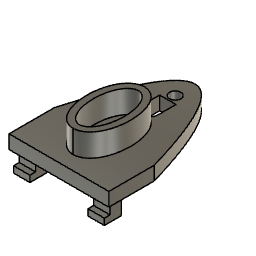
Here3 GPS Link Top Mount (Autodesk Fusion 360 design; units mm, degrees)
Autodesk Fusion 360 part; units mm, degrees
sketch "Sketch1" plane through (0, 0, 0) normal (0, 0, 1) x (1, 0, 0)
  line L0 (0, 0) -> (5.842, 0)
  line L1 (5.842, 0) -> (22.098, 0)
  line L2 (22.098, 0) -> (27.94, 0)
  line L3 (0, 0) -> (0, 12.7)
  line L4 (27.94, 0) -> (27.94, 12.7)
  line L5 (0, 0) -> (13.97, 0)
  line L6 (13.97, 0) -> (13.97, 38.1)
  spline S0 degree 5 poles (0, 12.7) (0.5588, 14.6265) (1.6764, 18.3113) (3.3528, 23.3339) (5.588, 29.0044) (8.382, 34.2662) (11.176, 37.5384) (13.97, 38.6587) (16.764, 37.5384) (19.558, 34.2662) (22.352, 29.0044) (24.5872, 23.3339) (26.2636, 18.3113) (27.3812, 14.6265) (27.94, 12.7) knots 0 0 0 0 0 0 0.1 0.2 0.3 0.4 0.5 0.6 0.7 0.8 0.9 1 1 1 1 1 1
  dimension "d1" = 5.842
  dimension "d2" = 16.256
  dimension "d3" = 5.842
  dimension "d28" = 13.97
  dimension "d29" = 38.1
  constraint coincident L0.start L3.start
  constraint horizontal L0
  constraint parallel L0 L1
  constraint parallel L1 L2
  constraint perpendicular L0 L3
  constraint perpendicular L2 L4
  constraint perpendicular L3 L5
  constraint perpendicular L5 L6
  measures "d1" distance of L0.start L0.end
  measures "d2" distance of L0.end L1.end
  measures "d3" distance of L1.end L2.end
  measures "d28" distance of L0.start L5.end
  measures "d29" distance of L5.end L6.end
extrude "Extrude1" add sketch "Sketch1" along normal blind 6.35
extrude "Extrude2" cut 1 faces at (13.0371, 11.4003, 6.35) along direction (0, 0, -1) blind 2.54
sketch "Sketch2" plane through (0, 0, 0) normal (0, 1, 0) x (1, 0, 0)
  line L0 (5.842, 0) -> (22.098, 0)
  line L1 (5.842, 0) -> (1.27, 0)
  line L2 (22.098, 0) -> (26.67, 0)
  line L3 (1.27, 0) -> (1.27, 5.08)
  line L4 (1.27, 5.08) -> (5.842, 5.08)
  line L5 (5.842, 0) -> (5.842, 5.08)
  line L6 (26.67, 0) -> (26.67, 5.08)
  line L7 (26.67, 5.08) -> (22.098, 5.08)
  line L8 (22.098, 5.08) -> (22.098, 0)
  line L9 (1.27, 0) -> (1.27, 3.302)
  line L10 (1.27, 3.302) -> (5.842, 3.302)
  line L11 (5.842, 0) -> (1.27, 0)
  line L12 (22.098, 0) -> (22.098, 3.302)
  line L13 (22.098, 3.302) -> (26.67, 3.302)
  line L14 (26.67, 0) -> (26.67, 3.302)
  line L15 (22.098, 0) -> (26.67, 0)
  dimension "d13" = 16.256
  dimension "d14" = 4.572
  dimension "d15" = 4.572
  dimension "d16" = 4.572
  dimension "d17" = 3.302
  dimension "d18" = 3.302
  constraint parallel L0 L1
  constraint parallel L0 L2
  constraint perpendicular L1 L3
  constraint perpendicular L3 L4
  constraint perpendicular L4 L5
  constraint perpendicular L2 L6
  constraint perpendicular L6 L7
  constraint perpendicular L2 L8
  constraint coincident L3 L9.end
  constraint coincident L5 L10.end
  constraint perpendicular L5 L10
  constraint coincident L8 L12.end
  constraint coincident L6 L13.end
  constraint perpendicular L12 L13
  measures "d13" distance of L0.start L0.end
  measures "d14" distance of L0.start L1.end
  measures "d15" distance of L0.end L2.end
  measures "d16" distance of L3.end L4.end
  measures "d17" distance of L1.end L9.end
  measures "d18" distance of L0.end L12.end
extrude "Extrude3" add sketch "Sketch2" along normal blind 3.175
sketch "Sketch3" plane through (0, 0, 0) normal (0, 1, 0) x (1, 0, 0)
  line L0 (1.27, 3.302) -> (5.842, 3.302)
  line L1 (5.842, 3.302) -> (5.842, 0)
  line L2 (5.842, 0) -> (1.27, 0)
  line L3 (1.27, 0) -> (1.27, 3.302)
  line L4 (22.098, 3.302) -> (22.098, 0)
  line L5 (22.098, 0) -> (26.67, 0)
  line L6 (26.67, 0) -> (26.67, 3.302)
  line L7 (26.67, 3.302) -> (22.098, 3.302)
  dimension "d22" = 4.572
  dimension "d23" = 16.256
  constraint perpendicular L0 L1
  constraint perpendicular L1 L2
  constraint perpendicular L2 L3
  constraint perpendicular L4 L5
  constraint perpendicular L4 L7
  measures "d22" distance of L0.start L0.end
  measures "d23" distance of L0.end L4.start
extrude "Extrude4" cut sketch "Sketch3" along normal blind 1.5875
extrude "Extrude5" add 2 faces at (23.622, 3.175, -3.3867) (4.318, 3.175, -3.3867) along direction (0, 1, 0) blind 1.5875
sketch "Sketch4" plane through (0, 0, 3.81) normal (0, 0, 1) x (-1, 0, 0)
  line L0 (0, 0) -> (-27.94, 0)
  line L1 (-27.94, 0) -> (-27.94, -12.7)
  line L2 (0, -12.7) -> (0, 0)
  spline S0 degree 3 poles (0, -12.7) (-2.8965, -22.686) (-5.7849, -30.0078) (-9.3219, -35.1431) (-10.13, -36.1462) (-11.5168, -37.2829) (-12.0485, -37.6254) (-13.0688, -38.0127) (-13.5272, -38.104) (-14.5137, -38.0954) (-15.0062, -37.9793) (-16.1808, -37.4795) (-16.8176, -37.0003) (-18.4204, -35.4814) (-19.6029, -33.9267) (-23.6727, -26.3115) (-26.0853, -19.0943) (-27.94, -12.7) knots -8.914263 -8.914263 -8.914263 -8.914263 -5.422922 -5.422922 -4.615305 -4.615305 -4.191653 -4.191653 -3.866732 -3.866732 -3.515116 -3.515116 -2.991073 -2.991073 -1.997365 -1.997365 0 0 0 0
  line L3 (0, 0) -> (-13.97, 0)
  circle A0 centre (-13.97, -32.5437) radius 1.5875
  line L4 (0, 0) -> (-13.97, 0)
  line L5 (-13.97, 0) -> (-13.97, -13.97)
  ellipse E0 centre (-13.97, -13.97) end of major axis (-13.97, -22.225) minor radius 4.318
  line L6 (-13.97, -5.715) -> (-13.97, -22.225)
  line L7 (-18.288, -13.97) -> (-9.652, -13.97)
  spline S1 degree 3 poles (-13.97, -3.937) (-15.0586, -3.937) (-16.097, -4.4015) (-16.9033, -5.0958) (-18.3617, -6.3515) (-19.2511, -8.3125) (-19.7163, -10.5249) (-20.3993, -13.7728) (-20.0754, -17.5624) (-18.7583, -20.3126) (-18.1661, -21.5491) (-17.3753, -22.6042) (-16.3066, -23.2908) (-15.4536, -23.8389) (-14.3857, -24.1121) (-13.3626, -23.9571) (-12.2174, -23.7837) (-11.2212, -23.1294) (-10.4581, -22.2736) (-9.0231, -20.6642) (-8.2215, -18.2814) (-7.9619, -15.7192) (-7.6924, -13.0599) (-8.0462, -10.2383) (-9.0065, -8.0127) (-9.5685, -6.7101) (-10.3321, -5.5893) (-11.3777, -4.8247) (-12.1184, -4.283) (-13.0302, -3.937) (-13.97, -3.937) knots -3.141593 -3.141593 -3.141593 -3.141593 -2.718421 -2.718421 -2.718421 -1.953052 -1.953052 -1.953052 -0.829428 -0.829428 -0.829428 -0.324215 -0.324215 -0.324215 0.079075 0.079075 0.079075 0.530523 0.530523 0.530523 1.379451 1.379451 1.379451 2.260522 2.260522 2.260522 2.776233 2.776233 2.776233 3.141593 3.141593 3.141593 3.141593
  dimension "d31" = 3.175
  dimension "d32" = 13.97
  dimension "d33" = 16.51
  dimension "d34" = 8.636
  dimension "d35" = 1.778
  constraint coincident L0.start L2.end
  constraint midpoint L0 L3.end
  constraint perpendicular L4 L5
  constraint coincident L5.end E0.centre
  constraint parallel L5 L6
  constraint coincident E0 L6.start
  constraint coincident E0 L6.end
  constraint coincident E0 L7.start
  constraint coincident E0 L7.end
  measures "d31" diameter of A0
  measures "d32" distance of L3.end L5.end
  measures "d33" distance of E0
extrude "Extrude6" add sketch "Sketch4" along normal blind 6.35 contours S1
sketch "Sketch5" plane through (0, 0, 3.81) normal (0, 0, 1) x (1, 0, 0)
  line L0 (0, 0) -> (13.97, 0)
  circle A0 centre (13.97, 32.5438) radius 1.5875
  line L1 (13.97, 32.5438) -> (13.97, 38.1)
  line L2 (11.684, 25.4) -> (11.684, 30.48)
  line L3 (11.684, 30.48) -> (16.256, 30.48)
  line L4 (16.256, 30.48) -> (16.256, 29.6684)
  line L5 (16.256, 29.6684) -> (16.256, 25.4)
  arc A1 (11.684, 25.4) -> (16.256, 25.4) centre (13.97, 25.4) ccw
  dimension "d38" = 13.97
  dimension "d40" = 3.175
  dimension "d46" = 4.572
  constraint coincident L0.start origin
  constraint horizontal L0
  constraint coincident A0.centre L1.start
  constraint vertical L1
  constraint vertical L2
  constraint perpendicular L2 L3
  constraint perpendicular L3 L4
  constraint perpendicular L3 L5
  constraint tangent L5 A1
  measures "d38" distance of L0.start L0.end
  measures "d40" diameter of A0
  measures "d46" distance of L2.end L3.end
extrude "Extrude7" cut sketch "Sketch5" against normal blind 12.7 contours A0
extrude "Extrude8" cut sketch "Sketch5" against normal blind 5.08 contours L2 L3 L4 L5 A1
